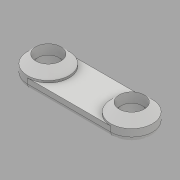
# Autodesk Inventor part: Link_1
Saved by Autodesk Inventor 2020 (Build 240168000, 168)
## iProperties
Created: 2020-02-22
Part Number: Link_1
Material: Generic
Document SubType Name: Modeling
Designer: Pece Jovanovski
Density: 1 g/cm^3
Appearance: Default
Mass: 0.0047854 g
Surface Area: 0.294248 cm^2
Volume: 0.0047854 cm^3
Author: Pece Jovanovski
Autodesk Inventor part; units mm, degrees
ref_plane "YZ Plane" through (0, 0, 0) normal (1, 0, 0) x (0, 1, 0)
ref_plane "XZ Plane" through (0, 0, 0) normal (0, 1, 0) x (-1, 0, 0)
ref_plane "XY Plane" through (0, 0, 0) normal (0, 0, 1) x (1, 0, 0)
sketch "Sketch1" plane through (0, 0, 0) normal (0, 0, 1) x (1, 0, 0)
  line L0 (-3, 1) -> (3, 1)
  line L1 (3, 1) -> (3, -1)
  line L2 (3, -1) -> (-3, -1)
  line L3 (-3, -1) -> (-3, 1)
  circle A0 centre (-2, 0) radius 0.5
  circle A1 centre (2, 0) radius 0.5
  point P0 (0, 0)
  point P1 (-3, 0)
  point P2 (0, 1)
  dimension "d0" = 6
  dimension "d1" = 2
  dimension "d2" = 1
  dimension "d3" = 1
  dimension "d4" = 4
  dimension "d5" = 2
  constraints: 8 end point, 3 horizontal alignment, 2 centre point, 2 midpoint, 2 parallel, 1 horizontal, 1 perpendicular, 1 vertical alignment
  measures "d0" distance between parallel lines of L1 L3
  measures "d1" distance between parallel lines of L2 L0
  measures "d2" diameter of A0
  measures "d3" diameter of A1
  measures "d4" distance of A1.centre A0.centre
  measures "d5" distance of point (0, 0) A0.centre
extrude "Extrusion1" add sketch "Sketch1" along normal mid plane 0.5
fillet "Fillet1" radius 1 4 edges at (3, 1, 0) (3, -1, 0) (-3, 1, 0) (-3, -1, 0)
sketch "Sketch2" plane through (0, 0, 0.25) normal (0, 0, 1) x (1, 0, 0)
  circle A0 centre (-2, 0) radius 0.5 projected
  circle A1 centre (-2, 0) radius 0.6
  circle A2 centre (2, 0) radius 0.5 projected
  circle A3 centre (2, 0) radius 0.6
  circle A4 centre (2, 0) radius 1
  circle A5 centre (-2, 0) radius 1
  point P0 (0, 0)
  dimension "d9" = 1.2
  dimension "d15" = 1.2
  dimension "d21" = 2
  dimension "d22" = 2
  constraints: 4 centre point, 4 coincident
  measures "d9" diameter of A1
  measures "d15" diameter of A3
  measures "d21" diameter of A4
  measures "d22" diameter of A5
extrude "Extrusion2" add sketch "Sketch2" along normal blind 0.1 contours A1
chamfer "Chamfer1" distance 0.1 angle 45 1 edges at (-2.6, 0, 0.35)
extrude "Extrusion3" add sketch "Sketch2" along normal blind 0.1 contours A3
chamfer "Chamfer2" distance 0.1 angle 45 1 edges at (1.4, 0, 0.35)
extrude "Extrusion4" add sketch "Sketch2" along normal blind 0.5 contours A4 | A5
chamfer "Chamfer3" distance 0.4 angle 45 2 edges at (1, 0, 0.75) (-3, 0, 0.75)
fillet "Fillet2" radius 0.25 8 edges at (-2.7071, 0.7071, -0.25) (-3, 0, -0.25) (-2.7071, -0.7071, -0.25) (0, 1, -0.25) (2.7071, -0.7071, -0.25) (2.7071, 0.7071, -0.25) (3, 0, -0.25) (0, -1, -0.25)
chamfer "Chamfer4" distance 0.15 angle 45 1 edges at (-2.5, 0, -0.25)
body "Solid1"
